增高架 (Autodesk Fusion 360 design; units mm, degrees)
part number: 2026-05-03-09-00-51-112
Autodesk Fusion 360 part; units mm, degrees
(part 1 of 4)
sketch "草图1" plane through (0, 0, 0) normal (0, 0, 1) x (1, 0, 0)
  line L0 (62.5, -90) -> (62.5, 85) construction
  line L1 (57.5, 90) -> (-57.5, 90) construction
  line L2 (-62.5, 85) -> (-62.5, -90) construction
  line L3 (-62.5, -90) -> (62.5, 90) construction
  line L4 (62.5, -90) -> (-62.5, 90) construction
  arc A0 (-57.5, 90) -> (-62.5, 85) centre (-57.5, 85) ccw construction
  arc A1 (62.5, 85) -> (57.5, 90) centre (57.5, 85) ccw construction
  line L5 (64, -90) -> (64, 85)
  arc A2 (64, 85) -> (57.5, 91.5) centre (57.5, 85) ccw
  line L6 (57.5, 91.5) -> (-57.5, 91.5)
  arc A3 (-57.5, 91.5) -> (-64, 85) centre (-57.5, 85) ccw
  line L7 (-64, 85) -> (-64, -90)
  line L8 (61, -90) -> (61, 85)
  arc A4 (61, 85) -> (57.5, 88.5) centre (57.5, 85) ccw
  line L9 (57.5, 88.5) -> (-57.5, 88.5)
  arc A5 (-57.5, 88.5) -> (-61, 85) centre (-57.5, 85) ccw
  line L10 (-61, 85) -> (-61, -90)
  line L11 (-64, -90) -> (-61, -90)
  line L12 (61, -90) -> (64, -90)
  line L13 (60.2436, 25.7321) -> (68.9038, 20.7321)
  dimension "d1" = 125
  dimension "d3" = 180
  dimension "d4" = 5
  dimension "d5" = 5
  dimension "d6" = 1.5
  dimension "d7" = -1.5
  constraint parallel L0 L2
  constraint coincident L3 origin
  constraint coincident L4 origin
  constraint horizontal L1
  constraint vertical L2
  constraint coincident L4.end L1
  constraint coincident L4.end L2
  constraint tangent L1 A0
  constraint tangent L2 A0
  constraint coincident L3.end L1
  constraint coincident L3.end L0
  constraint tangent L1 A1
  constraint tangent L0 A1
  constraint perpendicular L10 L11
  constraint perpendicular L5 L12
  measures "d1" distance of L0 L2
  measures "d3" distance of L2.end L4.end
  measures "d4" radius of A0
  measures "d5" radius of A1
extrude "拉伸1" add sketch "草图1" along normal blind 250
sketch "草图4" plane through (0, 91.5, 0) normal (0, 1, 0) x (-1, 0, 0)
  line L0 (-57.5, 0) -> (57.5, 0)
  line L1 (57.5, 0) -> (57.5, 250)
  line L2 (57.5, 250) -> (-57.5, 250)
  line L3 (-57.5, 250) -> (-57.5, 0)
  line L4 (48.5, 14) -> (44.1699, 11.5)
  line L5 (44.1699, 11.5) -> (44.1699, 6.5)
  line L6 (44.1699, 6.5) -> (48.5, 4)
  line L7 (48.5, 4) -> (52.8301, 6.5)
  line L8 (52.8301, 6.5) -> (52.8301, 11.5)
  line L9 (52.8301, 11.5) -> (48.5, 14)
  line L10 (37.8397, 14) -> (33.5096, 11.5)
  line L11 (33.5096, 11.5) -> (33.5096, 6.5)
  line L12 (33.5096, 6.5) -> (37.8397, 4)
  line L13 (37.8397, 4) -> (42.1699, 6.5)
  line L14 (42.1699, 6.5) -> (42.1699, 11.5)
  line L15 (42.1699, 11.5) -> (37.8397, 14)
  line L16 (27.1795, 14) -> (22.8494, 11.5)
  line L17 (22.8494, 11.5) -> (22.8494, 6.5)
  line L18 (22.8494, 6.5) -> (27.1795, 4)
  line L19 (27.1795, 4) -> (31.5096, 6.5)
  line L20 (31.5096, 6.5) -> (31.5096, 11.5)
  line L21 (31.5096, 11.5) -> (27.1795, 14)
  line L22 (16.5192, 14) -> (12.1891, 11.5)
  line L23 (12.1891, 11.5) -> (12.1891, 6.5)
  line L24 (12.1891, 6.5) -> (16.5192, 4)
  line L25 (16.5192, 4) -> (20.8494, 6.5)
  line L26 (20.8494, 6.5) -> (20.8494, 11.5)
  line L27 (20.8494, 11.5) -> (16.5192, 14)
  line L28 (5.859, 14) -> (1.5289, 11.5)
  line L29 (1.5289, 11.5) -> (1.5289, 6.5)
  line L30 (1.5289, 6.5) -> (5.859, 4)
  line L31 (5.859, 4) -> (10.1891, 6.5)
  line L32 (10.1891, 6.5) -> (10.1891, 11.5)
  line L33 (10.1891, 11.5) -> (5.859, 14)
  line L34 (-4.8013, 14) -> (-9.1314, 11.5)
  line L35 (-9.1314, 11.5) -> (-9.1314, 6.5)
  line L36 (-9.1314, 6.5) -> (-4.8013, 4)
  line L37 (-4.8013, 4) -> (-0.4711, 6.5)
  line L38 (-0.4711, 6.5) -> (-0.4711, 11.5)
  line L39 (-0.4711, 11.5) -> (-4.8013, 14)
  line L40 (-15.4615, 14) -> (-19.7917, 11.5)
  line L41 (-19.7917, 11.5) -> (-19.7917, 6.5)
  line L42 (-19.7917, 6.5) -> (-15.4615, 4)
  line L43 (-15.4615, 4) -> (-11.1314, 6.5)
  line L44 (-11.1314, 6.5) -> (-11.1314, 11.5)
  line L45 (-11.1314, 11.5) -> (-15.4615, 14)
  line L46 (-26.1218, 14) -> (-30.4519, 11.5)
  line L47 (-30.4519, 11.5) -> (-30.4519, 6.5)
  line L48 (-30.4519, 6.5) -> (-26.1218, 4)
  line L49 (-26.1218, 4) -> (-21.7917, 6.5)
  line L50 (-21.7917, 6.5) -> (-21.7917, 11.5)
  line L51 (-21.7917, 11.5) -> (-26.1218, 14)
  line L52 (-36.782, 14) -> (-41.1122, 11.5)
  line L53 (-41.1122, 11.5) -> (-41.1122, 6.5)
  line L54 (-41.1122, 6.5) -> (-36.782, 4)
  line L55 (-36.782, 4) -> (-32.4519, 6.5)
  line L56 (-32.4519, 6.5) -> (-32.4519, 11.5)
  line L57 (-32.4519, 11.5) -> (-36.782, 14)
  line L58 (-47.4423, 14) -> (-51.7724, 11.5)
  line L59 (-51.7724, 11.5) -> (-51.7724, 6.5)
  line L60 (-51.7724, 6.5) -> (-47.4423, 4)
  line L61 (-47.4423, 4) -> (-43.1122, 6.5)
  line L62 (-43.1122, 6.5) -> (-43.1122, 11.5)
  line L63 (-43.1122, 11.5) -> (-47.4423, 14)
  line L64 (43.1699, 23.2321) -> (38.8397, 20.7321)
  line L65 (38.8397, 20.7321) -> (38.8397, 15.7321)
  line L66 (38.8397, 15.7321) -> (43.1699, 13.2321)
  line L67 (43.1699, 13.2321) -> (47.5, 15.7321)
  line L68 (47.5, 15.7321) -> (47.5, 20.7321)
  line L69 (47.5, 20.7321) -> (43.1699, 23.2321)
  line L70 (32.5096, 23.2321) -> (28.1795, 20.7321)
  line L71 (28.1795, 20.7321) -> (28.1795, 15.7321)
  line L72 (28.1795, 15.7321) -> (32.5096, 13.2321)
  line L73 (32.5096, 13.2321) -> (36.8397, 15.7321)
  line L74 (36.8397, 15.7321) -> (36.8397, 20.7321)
  line L75 (36.8397, 20.7321) -> (32.5096, 23.2321)
  line L76 (21.8494, 23.2321) -> (17.5192, 20.7321)
  line L77 (17.5192, 20.7321) -> (17.5192, 15.7321)
  line L78 (17.5192, 15.7321) -> (21.8494, 13.2321)
  line L79 (21.8494, 13.2321) -> (26.1795, 15.7321)
  line L80 (26.1795, 15.7321) -> (26.1795, 20.7321)
  line L81 (26.1795, 20.7321) -> (21.8494, 23.2321)
  line L82 (11.1891, 23.2321) -> (6.859, 20.7321)
  line L83 (6.859, 20.7321) -> (6.859, 15.7321)
  line L84 (6.859, 15.7321) -> (11.1891, 13.2321)
  line L85 (11.1891, 13.2321) -> (15.5192, 15.7321)
  line L86 (15.5192, 15.7321) -> (15.5192, 20.7321)
  line L87 (15.5192, 20.7321) -> (11.1891, 23.2321)
  line L88 (0.5289, 23.2321) -> (-3.8013, 20.7321)
  line L89 (-3.8013, 20.7321) -> (-3.8013, 15.7321)
  line L90 (-3.8013, 15.7321) -> (0.5289, 13.2321)
  line L91 (0.5289, 13.2321) -> (4.859, 15.7321)
  line L92 (4.859, 15.7321) -> (4.859, 20.7321)
  line L93 (4.859, 20.7321) -> (0.5289, 23.2321)
  line L94 (-10.1314, 23.2321) -> (-14.4615, 20.7321)
  line L95 (-14.4615, 20.7321) -> (-14.4615, 15.7321)
  line L96 (-14.4615, 15.7321) -> (-10.1314, 13.2321)
  line L97 (-10.1314, 13.2321) -> (-5.8013, 15.7321)
  line L98 (-5.8013, 15.7321) -> (-5.8013, 20.7321)
  line L99 (-5.8013, 20.7321) -> (-10.1314, 23.2321)
  line L100 (-20.7917, 23.2321) -> (-25.1218, 20.7321)
  line L101 (-25.1218, 20.7321) -> (-25.1218, 15.7321)
  line L102 (-25.1218, 15.7321) -> (-20.7917, 13.2321)
  line L103 (-20.7917, 13.2321) -> (-16.4615, 15.7321)
  line L104 (-16.4615, 15.7321) -> (-16.4615, 20.7321)
  line L105 (-16.4615, 20.7321) -> (-20.7917, 23.2321)
  line L106 (-31.4519, 23.2321) -> (-35.782, 20.7321)
  line L107 (-35.782, 20.7321) -> (-35.782, 15.7321)
  line L108 (-35.782, 15.7321) -> (-31.4519, 13.2321)
  line L109 (-31.4519, 13.2321) -> (-27.1218, 15.7321)
  line L110 (-27.1218, 15.7321) -> (-27.1218, 20.7321)
  line L111 (-27.1218, 20.7321) -> (-31.4519, 23.2321)
  line L112 (-42.1122, 23.2321) -> (-46.4423, 20.7321)
  line L113 (-46.4423, 20.7321) -> (-46.4423, 15.7321)
  line L114 (-46.4423, 15.7321) -> (-42.1122, 13.2321)
  line L115 (-42.1122, 13.2321) -> (-37.782, 15.7321)
  line L116 (-37.782, 15.7321) -> (-37.782, 20.7321)
  line L117 (-37.782, 20.7321) -> (-42.1122, 23.2321)
  line L118 (48.5, 32.4641) -> (44.1699, 29.9641)
  line L119 (44.1699, 29.9641) -> (44.1699, 24.9641)
  line L120 (44.1699, 24.9641) -> (48.5, 22.4641)
  line L121 (48.5, 22.4641) -> (52.8301, 24.9641)
  line L122 (52.8301, 24.9641) -> (52.8301, 29.9641)
  line L123 (52.8301, 29.9641) -> (48.5, 32.4641)
  line L124 (37.8397, 32.4641) -> (33.5096, 29.9641)
  line L125 (33.5096, 29.9641) -> (33.5096, 24.9641)
  line L126 (33.5096, 24.9641) -> (37.8397, 22.4641)
  line L127 (37.8397, 22.4641) -> (42.1699, 24.9641)
  line L128 (42.1699, 24.9641) -> (42.1699, 29.9641)
  line L129 (42.1699, 29.9641) -> (37.8397, 32.4641)
  line L130 (27.1795, 32.4641) -> (22.8494, 29.9641)
  line L131 (22.8494, 29.9641) -> (22.8494, 24.9641)
  line L132 (22.8494, 24.9641) -> (27.1795, 22.4641)
  line L133 (27.1795, 22.4641) -> (31.5096, 24.9641)
  line L134 (31.5096, 24.9641) -> (31.5096, 29.9641)
  line L135 (31.5096, 29.9641) -> (27.1795, 32.4641)
  line L136 (16.5192, 32.4641) -> (12.1891, 29.9641)
  line L137 (12.1891, 29.9641) -> (12.1891, 24.9641)
  line L138 (12.1891, 24.9641) -> (16.5192, 22.4641)
  line L139 (16.5192, 22.4641) -> (20.8494, 24.9641)
  line L140 (20.8494, 24.9641) -> (20.8494, 29.9641)
  line L141 (20.8494, 29.9641) -> (16.5192, 32.4641)
  line L142 (5.859, 32.4641) -> (1.5289, 29.9641)
  line L143 (1.5289, 29.9641) -> (1.5289, 24.9641)
  line L144 (1.5289, 24.9641) -> (5.859, 22.4641)
  line L145 (5.859, 22.4641) -> (10.1891, 24.9641)
  line L146 (10.1891, 24.9641) -> (10.1891, 29.9641)
  line L147 (10.1891, 29.9641) -> (5.859, 32.4641)
  line L148 (-4.8013, 32.4641) -> (-9.1314, 29.9641)
  line L149 (-9.1314, 29.9641) -> (-9.1314, 24.9641)
  line L150 (-9.1314, 24.9641) -> (-4.8013, 22.4641)
  line L151 (-4.8013, 22.4641) -> (-0.4711, 24.9641)
  line L152 (-0.4711, 24.9641) -> (-0.4711, 29.9641)
  line L153 (-0.4711, 29.9641) -> (-4.8013, 32.4641)
  line L154 (-15.4615, 32.4641) -> (-19.7917, 29.9641)
  line L155 (-19.7917, 29.9641) -> (-19.7917, 24.9641)
  line L156 (-19.7917, 24.9641) -> (-15.4615, 22.4641)
  line L157 (-15.4615, 22.4641) -> (-11.1314, 24.9641)
  line L158 (-11.1314, 24.9641) -> (-11.1314, 29.9641)
  line L159 (-11.1314, 29.9641) -> (-15.4615, 32.4641)
  line L160 (-26.1218, 32.4641) -> (-30.4519, 29.9641)
  line L161 (-30.4519, 29.9641) -> (-30.4519, 24.9641)
  line L162 (-30.4519, 24.9641) -> (-26.1218, 22.4641)
  line L163 (-26.1218, 22.4641) -> (-21.7917, 24.9641)
  line L164 (-21.7917, 24.9641) -> (-21.7917, 29.9641)
  line L165 (-21.7917, 29.9641) -> (-26.1218, 32.4641)
  line L166 (-36.782, 32.4641) -> (-41.1122, 29.9641)
  line L167 (-41.1122, 29.9641) -> (-41.1122, 24.9641)
  line L168 (-41.1122, 24.9641) -> (-36.782, 22.4641)
  line L169 (-36.782, 22.4641) -> (-32.4519, 24.9641)
  line L170 (-32.4519, 24.9641) -> (-32.4519, 29.9641)
  line L171 (-32.4519, 29.9641) -> (-36.782, 32.4641)
  line L172 (-47.4423, 32.4641) -> (-51.7724, 29.9641)
  line L173 (-51.7724, 29.9641) -> (-51.7724, 24.9641)
  line L174 (-51.7724, 24.9641) -> (-47.4423, 22.4641)
  line L175 (-47.4423, 22.4641) -> (-43.1122, 24.9641)
  line L176 (-43.1122, 24.9641) -> (-43.1122, 29.9641)
  line L177 (-43.1122, 29.9641) -> (-47.4423, 32.4641)
  line L178 (43.1699, 41.6962) -> (38.8397, 39.1962)
  line L179 (38.8397, 39.1962) -> (38.8397, 34.1962)
  line L180 (38.8397, 34.1962) -> (43.1699, 31.6962)
  line L181 (43.1699, 31.6962) -> (47.5, 34.1962)
  line L182 (47.5, 34.1962) -> (47.5, 39.1962)
  line L183 (47.5, 39.1962) -> (43.1699, 41.6962)
  line L184 (32.5096, 41.6962) -> (28.1795, 39.1962)
  line L185 (28.1795, 39.1962) -> (28.1795, 34.1962)
  line L186 (28.1795, 34.1962) -> (32.5096, 31.6962)
  line L187 (32.5096, 31.6962) -> (36.8397, 34.1962)
  line L188 (36.8397, 34.1962) -> (36.8397, 39.1962)
  line L189 (36.8397, 39.1962) -> (32.5096, 41.6962)
  line L190 (21.8494, 41.6962) -> (17.5192, 39.1962)
  line L191 (17.5192, 39.1962) -> (17.5192, 34.1962)
  line L192 (17.5192, 34.1962) -> (21.8494, 31.6962)
  line L193 (21.8494, 31.6962) -> (26.1795, 34.1962)
  line L194 (26.1795, 34.1962) -> (26.1795, 39.1962)
  line L195 (26.1795, 39.1962) -> (21.8494, 41.6962)
  line L196 (11.1891, 41.6962) -> (6.859, 39.1962)
  line L197 (6.859, 39.1962) -> (6.859, 34.1962)
  line L198 (6.859, 34.1962) -> (11.1891, 31.6962)
  line L199 (11.1891, 31.6962) -> (15.5192, 34.1962)
  line L200 (15.5192, 34.1962) -> (15.5192, 39.1962)
  line L201 (15.5192, 39.1962) -> (11.1891, 41.6962)
  line L202 (0.5289, 41.6962) -> (-3.8013, 39.1962)
  line L203 (-3.8013, 39.1962) -> (-3.8013, 34.1962)
  line L204 (-3.8013, 34.1962) -> (0.5289, 31.6962)
  line L205 (0.5289, 31.6962) -> (4.859, 34.1962)
  line L206 (4.859, 34.1962) -> (4.859, 39.1962)
  line L207 (4.859, 39.1962) -> (0.5289, 41.6962)
  line L208 (-10.1314, 41.6962) -> (-14.4615, 39.1962)
  line L209 (-14.4615, 39.1962) -> (-14.4615, 34.1962)
  line L210 (-14.4615, 34.1962) -> (-10.1314, 31.6962)
  line L211 (-10.1314, 31.6962) -> (-5.8013, 34.1962)
  line L212 (-5.8013, 34.1962) -> (-5.8013, 39.1962)
  line L213 (-5.8013, 39.1962) -> (-10.1314, 41.6962)
  line L214 (-20.7917, 41.6962) -> (-25.1218, 39.1962)
  line L215 (-25.1218, 39.1962) -> (-25.1218, 34.1962)
  line L216 (-25.1218, 34.1962) -> (-20.7917, 31.6962)
  line L217 (-20.7917, 31.6962) -> (-16.4615, 34.1962)
  line L218 (-16.4615, 34.1962) -> (-16.4615, 39.1962)
  line L219 (-16.4615, 39.1962) -> (-20.7917, 41.6962)
  line L220 (-31.4519, 41.6962) -> (-35.782, 39.1962)
  line L221 (-35.782, 39.1962) -> (-35.782, 34.1962)
  line L222 (-35.782, 34.1962) -> (-31.4519, 31.6962)
  line L223 (-31.4519, 31.6962) -> (-27.1218, 34.1962)
  line L224 (-27.1218, 34.1962) -> (-27.1218, 39.1962)
  line L225 (-27.1218, 39.1962) -> (-31.4519, 41.6962)
  line L226 (-42.1122, 41.6962) -> (-46.4423, 39.1962)
  line L227 (-46.4423, 39.1962) -> (-46.4423, 34.1962)
  line L228 (-46.4423, 34.1962) -> (-42.1122, 31.6962)
  line L229 (-42.1122, 31.6962) -> (-37.782, 34.1962)
  line L230 (-37.782, 34.1962) -> (-37.782, 39.1962)
  line L231 (-37.782, 39.1962) -> (-42.1122, 41.6962)
  line L232 (48.5, 50.9282) -> (44.1699, 48.4282)
  line L233 (44.1699, 48.4282) -> (44.1699, 43.4282)
  line L234 (44.1699, 43.4282) -> (48.5, 40.9282)
  line L235 (48.5, 40.9282) -> (52.8301, 43.4282)
  line L236 (52.8301, 43.4282) -> (52.8301, 48.4282)
  line L237 (52.8301, 48.4282) -> (48.5, 50.9282)
  line L238 (37.8397, 50.9282) -> (33.5096, 48.4282)
  line L239 (33.5096, 48.4282) -> (33.5096, 43.4282)
  line L240 (33.5096, 43.4282) -> (37.8397, 40.9282)
  line L241 (37.8397, 40.9282) -> (42.1699, 43.4282)
  line L242 (42.1699, 43.4282) -> (42.1699, 48.4282)
  line L243 (42.1699, 48.4282) -> (37.8397, 50.9282)
  line L244 (27.1795, 50.9282) -> (22.8494, 48.4282)
  line L245 (22.8494, 48.4282) -> (22.8494, 43.4282)
  line L246 (22.8494, 43.4282) -> (27.1795, 40.9282)
  line L247 (27.1795, 40.9282) -> (31.5096, 43.4282)
  line L248 (31.5096, 43.4282) -> (31.5096, 48.4282)
  line L249 (31.5096, 48.4282) -> (27.1795, 50.9282)
  line L250 (16.5192, 50.9282) -> (12.1891, 48.4282)
  line L251 (12.1891, 48.4282) -> (12.1891, 43.4282)
  line L252 (12.1891, 43.4282) -> (16.5192, 40.9282)
  line L253 (16.5192, 40.9282) -> (20.8494, 43.4282)
  line L254 (20.8494, 43.4282) -> (20.8494, 48.4282)
  line L255 (20.8494, 48.4282) -> (16.5192, 50.9282)
  line L256 (5.859, 50.9282) -> (1.5289, 48.4282)
  line L257 (1.5289, 48.4282) -> (1.5289, 43.4282)
  line L258 (1.5289, 43.4282) -> (5.859, 40.9282)
  line L259 (5.859, 40.9282) -> (10.1891, 43.4282)
  line L260 (10.1891, 43.4282) -> (10.1891, 48.4282)
  line L261 (10.1891, 48.4282) -> (5.859, 50.9282)
  line L262 (-4.8013, 50.9282) -> (-9.1314, 48.4282)
  line L263 (-9.1314, 48.4282) -> (-9.1314, 43.4282)
  line L264 (-9.1314, 43.4282) -> (-4.8013, 40.9282)
  line L265 (-4.8013, 40.9282) -> (-0.4711, 43.4282)
  line L266 (-0.4711, 43.4282) -> (-0.4711, 48.4282)
  line L267 (-0.4711, 48.4282) -> (-4.8013, 50.9282)
  line L268 (-15.4615, 50.9282) -> (-19.7917, 48.4282)
  line L269 (-19.7917, 48.4282) -> (-19.7917, 43.4282)
  line L270 (-19.7917, 43.4282) -> (-15.4615, 40.9282)
  line L271 (-15.4615, 40.9282) -> (-11.1314, 43.4282)
  line L272 (-11.1314, 43.4282) -> (-11.1314, 48.4282)
  line L273 (-11.1314, 48.4282) -> (-15.4615, 50.9282)
  line L274 (-26.1218, 50.9282) -> (-30.4519, 48.4282)
  line L275 (-30.4519, 48.4282) -> (-30.4519, 43.4282)
  line L276 (-30.4519, 43.4282) -> (-26.1218, 40.9282)
  line L277 (-26.1218, 40.9282) -> (-21.7917, 43.4282)
  line L278 (-21.7917, 43.4282) -> (-21.7917, 48.4282)
  line L279 (-21.7917, 48.4282) -> (-26.1218, 50.9282)
  line L280 (-36.782, 50.9282) -> (-41.1122, 48.4282)
  line L281 (-41.1122, 48.4282) -> (-41.1122, 43.4282)
  line L282 (-41.1122, 43.4282) -> (-36.782, 40.9282)
  line L283 (-36.782, 40.9282) -> (-32.4519, 43.4282)
  line L284 (-32.4519, 43.4282) -> (-32.4519, 48.4282)
  line L285 (-32.4519, 48.4282) -> (-36.782, 50.9282)
  line L286 (-47.4423, 50.9282) -> (-51.7724, 48.4282)
  line L287 (-51.7724, 48.4282) -> (-51.7724, 43.4282)
  line L288 (-51.7724, 43.4282) -> (-47.4423, 40.9282)
  line L289 (-47.4423, 40.9282) -> (-43.1122, 43.4282)
  line L290 (-43.1122, 43.4282) -> (-43.1122, 48.4282)
  line L291 (-43.1122, 48.4282) -> (-47.4423, 50.9282)
  line L292 (43.1699, 60.1603) -> (38.8397, 57.6603)
  line L293 (38.8397, 57.6603) -> (38.8397, 52.6603)
  line L294 (38.8397, 52.6603) -> (43.1699, 50.1603)
  line L295 (43.1699, 50.1603) -> (47.5, 52.6603)
  line L296 (47.5, 52.6603) -> (47.5, 57.6603)
  line L297 (47.5, 57.6603) -> (43.1699, 60.1603)
  line L298 (32.5096, 60.1603) -> (28.1795, 57.6603)
  line L299 (28.1795, 57.6603) -> (28.1795, 52.6603)
  line L300 (28.1795, 52.6603) -> (32.5096, 50.1603)
  line L301 (32.5096, 50.1603) -> (36.8397, 52.6603)
  line L302 (36.8397, 52.6603) -> (36.8397, 57.6603)
  line L303 (36.8397, 57.6603) -> (32.5096, 60.1603)
  line L304 (21.8494, 60.1603) -> (17.5192, 57.6603)
  line L305 (17.5192, 57.6603) -> (17.5192, 52.6603)
  line L306 (17.5192, 52.6603) -> (21.8494, 50.1603)
  line L307 (21.8494, 50.1603) -> (26.1795, 52.6603)
  line L308 (26.1795, 52.6603) -> (26.1795, 57.6603)
  line L309 (26.1795, 57.6603) -> (21.8494, 60.1603)
  line L310 (11.1891, 60.1603) -> (6.859, 57.6603)
  line L311 (6.859, 57.6603) -> (6.859, 52.6603)
  line L312 (6.859, 52.6603) -> (11.1891, 50.1603)
  line L313 (11.1891, 50.1603) -> (15.5192, 52.6603)
  line L314 (15.5192, 52.6603) -> (15.5192, 57.6603)
  line L315 (15.5192, 57.6603) -> (11.1891, 60.1603)
  line L316 (0.5289, 60.1603) -> (-3.8013, 57.6603)
  line L317 (-3.8013, 57.6603) -> (-3.8013, 52.6603)
  line L318 (-3.8013, 52.6603) -> (0.5289, 50.1603)
  line L319 (0.5289, 50.1603) -> (4.859, 52.6603)
  line L320 (4.859, 52.6603) -> (4.859, 57.6603)
  line L321 (4.859, 57.6603) -> (0.5289, 60.1603)
  line L322 (-10.1314, 60.1603) -> (-14.4615, 57.6603)
  line L323 (-14.4615, 57.6603) -> (-14.4615, 52.6603)
  line L324 (-14.4615, 52.6603) -> (-10.1314, 50.1603)
  line L325 (-10.1314, 50.1603) -> (-5.8013, 52.6603)
  line L326 (-5.8013, 52.6603) -> (-5.8013, 57.6603)
  line L327 (-5.8013, 57.6603) -> (-10.1314, 60.1603)
  line L328 (-20.7917, 60.1603) -> (-25.1218, 57.6603)
  line L329 (-25.1218, 57.6603) -> (-25.1218, 52.6603)
  line L330 (-25.1218, 52.6603) -> (-20.7917, 50.1603)
  line L331 (-20.7917, 50.1603) -> (-16.4615, 52.6603)
  line L332 (-16.4615, 52.6603) -> (-16.4615, 57.6603)
  line L333 (-16.4615, 57.6603) -> (-20.7917, 60.1603)
  line L334 (-31.4519, 60.1603) -> (-35.782, 57.6603)
  line L335 (-35.782, 57.6603) -> (-35.782, 52.6603)
  line L336 (-35.782, 52.6603) -> (-31.4519, 50.1603)
  line L337 (-31.4519, 50.1603) -> (-27.1218, 52.6603)
  line L338 (-27.1218, 52.6603) -> (-27.1218, 57.6603)
  line L339 (-27.1218, 57.6603) -> (-31.4519, 60.1603)
  line L340 (-42.1122, 60.1603) -> (-46.4423, 57.6603)
  line L341 (-46.4423, 57.6603) -> (-46.4423, 52.6603)
  line L342 (-46.4423, 52.6603) -> (-42.1122, 50.1603)
  line L343 (-42.1122, 50.1603) -> (-37.782, 52.6603)
  line L344 (-37.782, 52.6603) -> (-37.782, 57.6603)
  line L345 (-37.782, 57.6603) -> (-42.1122, 60.1603)
  line L346 (48.5, 69.3923) -> (44.1699, 66.8923)
  line L347 (44.1699, 66.8923) -> (44.1699, 61.8923)
  line L348 (44.1699, 61.8923) -> (48.5, 59.3923)
  line L349 (48.5, 59.3923) -> (52.8301, 61.8923)
  line L350 (52.8301, 61.8923) -> (52.8301, 66.8923)
  line L351 (52.8301, 66.8923) -> (48.5, 69.3923)
  line L352 (37.8397, 69.3923) -> (33.5096, 66.8923)
  line L353 (33.5096, 66.8923) -> (33.5096, 61.8923)
  line L354 (33.5096, 61.8923) -> (37.8397, 59.3923)
  line L355 (37.8397, 59.3923) -> (42.1699, 61.8923)
  line L356 (42.1699, 61.8923) -> (42.1699, 66.8923)
  line L357 (42.1699, 66.8923) -> (37.8397, 69.3923)
  line L358 (27.1795, 69.3923) -> (22.8494, 66.8923)
  line L359 (22.8494, 66.8923) -> (22.8494, 61.8923)
  line L360 (22.8494, 61.8923) -> (27.1795, 59.3923)
  line L361 (27.1795, 59.3923) -> (31.5096, 61.8923)
  line L362 (31.5096, 61.8923) -> (31.5096, 66.8923)
  line L363 (31.5096, 66.8923) -> (27.1795, 69.3923)
  line L364 (16.5192, 69.3923) -> (12.1891, 66.8923)
  line L365 (12.1891, 66.8923) -> (12.1891, 61.8923)
  line L366 (12.1891, 61.8923) -> (16.5192, 59.3923)
  line L367 (16.5192, 59.3923) -> (20.8494, 61.8923)
  line L368 (20.8494, 61.8923) -> (20.8494, 66.8923)
  line L369 (20.8494, 66.8923) -> (16.5192, 69.3923)
  line L370 (5.859, 69.3923) -> (1.5289, 66.8923)
  line L371 (1.5289, 66.8923) -> (1.5289, 61.8923)
  line L372 (1.5289, 61.8923) -> (5.859, 59.3923)
  line L373 (5.859, 59.3923) -> (10.1891, 61.8923)
  line L374 (10.1891, 61.8923) -> (10.1891, 66.8923)
  line L375 (10.1891, 66.8923) -> (5.859, 69.3923)
  line L376 (-4.8013, 69.3923) -> (-9.1314, 66.8923)
  line L377 (-9.1314, 66.8923) -> (-9.1314, 61.8923)
  line L378 (-9.1314, 61.8923) -> (-4.8013, 59.3923)
  line L379 (-4.8013, 59.3923) -> (-0.4711, 61.8923)
  line L380 (-0.4711, 61.8923) -> (-0.4711, 66.8923)
  line L381 (-0.4711, 66.8923) -> (-4.8013, 69.3923)
  line L382 (-15.4615, 69.3923) -> (-19.7917, 66.8923)
  line L383 (-19.7917, 66.8923) -> (-19.7917, 61.8923)
  line L384 (-19.7917, 61.8923) -> (-15.4615, 59.3923)
  line L385 (-15.4615, 59.3923) -> (-11.1314, 61.8923)
  line L386 (-11.1314, 61.8923) -> (-11.1314, 66.8923)
  line L387 (-11.1314, 66.8923) -> (-15.4615, 69.3923)
  line L388 (-26.1218, 69.3923) -> (-30.4519, 66.8923)
  line L389 (-30.4519, 66.8923) -> (-30.4519, 61.8923)
  line L390 (-30.4519, 61.8923) -> (-26.1218, 59.3923)
  line L391 (-26.1218, 59.3923) -> (-21.7917, 61.8923)
  line L392 (-21.7917, 61.8923) -> (-21.7917, 66.8923)
  line L393 (-21.7917, 66.8923) -> (-26.1218, 69.3923)
  line L394 (-36.782, 69.3923) -> (-41.1122, 66.8923)
  line L395 (-41.1122, 66.8923) -> (-41.1122, 61.8923)
  line L396 (-41.1122, 61.8923) -> (-36.782, 59.3923)
  line L397 (-36.782, 59.3923) -> (-32.4519, 61.8923)
  line L398 (-32.4519, 61.8923) -> (-32.4519, 66.8923)
  line L399 (-32.4519, 66.8923) -> (-36.782, 69.3923)
  line L400 (-47.4423, 69.3923) -> (-51.7724, 66.8923)
  line L401 (-51.7724, 66.8923) -> (-51.7724, 61.8923)
  line L402 (-51.7724, 61.8923) -> (-47.4423, 59.3923)
  line L403 (-47.4423, 59.3923) -> (-43.1122, 61.8923)
  line L404 (-43.1122, 61.8923) -> (-43.1122, 66.8923)
  line L405 (-43.1122, 66.8923) -> (-47.4423, 69.3923)
  line L406 (43.1699, 78.6244) -> (38.8397, 76.1244)
  line L407 (38.8397, 76.1244) -> (38.8397, 71.1244)
  line L408 (38.8397, 71.1244) -> (43.1699, 68.6244)
  line L409 (43.1699, 68.6244) -> (47.5, 71.1244)
  line L410 (47.5, 71.1244) -> (47.5, 76.1244)
  line L411 (47.5, 76.1244) -> (43.1699, 78.6244)
  line L412 (32.5096, 78.6244) -> (28.1795, 76.1244)
  line L413 (28.1795, 76.1244) -> (28.1795, 71.1244)
  line L414 (28.1795, 71.1244) -> (32.5096, 68.6244)
  line L415 (32.5096, 68.6244) -> (36.8397, 71.1244)
  line L416 (36.8397, 71.1244) -> (36.8397, 76.1244)
  line L417 (36.8397, 76.1244) -> (32.5096, 78.6244)
  line L418 (21.8494, 78.6244) -> (17.5192, 76.1244)
  line L419 (17.5192, 76.1244) -> (17.5192, 71.1244)
  line L420 (17.5192, 71.1244) -> (21.8494, 68.6244)
  line L421 (21.8494, 68.6244) -> (26.1795, 71.1244)
  line L422 (26.1795, 71.1244) -> (26.1795, 76.1244)
  line L423 (26.1795, 76.1244) -> (21.8494, 78.6244)
  line L424 (11.1891, 78.6244) -> (6.859, 76.1244)
  line L425 (6.859, 76.1244) -> (6.859, 71.1244)
  line L426 (6.859, 71.1244) -> (11.1891, 68.6244)
  line L427 (11.1891, 68.6244) -> (15.5192, 71.1244)
  line L428 (15.5192, 71.1244) -> (15.5192, 76.1244)
  line L429 (15.5192, 76.1244) -> (11.1891, 78.6244)
  line L430 (0.5289, 78.6244) -> (-3.8013, 76.1244)
  line L431 (-3.8013, 76.1244) -> (-3.8013, 71.1244)
  line L432 (-3.8013, 71.1244) -> (0.5289, 68.6244)
  line L433 (0.5289, 68.6244) -> (4.859, 71.1244)
  line L434 (4.859, 71.1244) -> (4.859, 76.1244)
  line L435 (4.859, 76.1244) -> (0.5289, 78.6244)
  line L436 (-10.1314, 78.6244) -> (-14.4615, 76.1244)
  line L437 (-14.4615, 76.1244) -> (-14.4615, 71.1244)
  line L438 (-14.4615, 71.1244) -> (-10.1314, 68.6244)
  line L439 (-10.1314, 68.6244) -> (-5.8013, 71.1244)
  line L440 (-5.8013, 71.1244) -> (-5.8013, 76.1244)
  line L441 (-5.8013, 76.1244) -> (-10.1314, 78.6244)
  line L442 (-20.7917, 78.6244) -> (-25.1218, 76.1244)
  line L443 (-25.1218, 76.1244) -> (-25.1218, 71.1244)
  line L444 (-25.1218, 71.1244) -> (-20.7917, 68.6244)
  line L445 (-20.7917, 68.6244) -> (-16.4615, 71.1244)
  line L446 (-16.4615, 71.1244) -> (-16.4615, 76.1244)
  line L447 (-16.4615, 76.1244) -> (-20.7917, 78.6244)
  line L448 (-31.4519, 78.6244) -> (-35.782, 76.1244)
  line L449 (-35.782, 76.1244) -> (-35.782, 71.1244)
  line L450 (-35.782, 71.1244) -> (-31.4519, 68.6244)
  line L451 (-31.4519, 68.6244) -> (-27.1218, 71.1244)
  line L452 (-27.1218, 71.1244) -> (-27.1218, 76.1244)
  line L453 (-27.1218, 76.1244) -> (-31.4519, 78.6244)
  line L454 (-42.1122, 78.6244) -> (-46.4423, 76.1244)
  line L455 (-46.4423, 76.1244) -> (-46.4423, 71.1244)
  line L456 (-46.4423, 71.1244) -> (-42.1122, 68.6244)
  line L457 (-42.1122, 68.6244) -> (-37.782, 71.1244)
  line L458 (-37.782, 71.1244) -> (-37.782, 76.1244)
  line L459 (-37.782, 76.1244) -> (-42.1122, 78.6244)
  line L460 (48.5, 87.8564) -> (44.1699, 85.3564)
  line L461 (44.1699, 85.3564) -> (44.1699, 80.3564)
  line L462 (44.1699, 80.3564) -> (48.5, 77.8564)
  line L463 (48.5, 77.8564) -> (52.8301, 80.3564)
  line L464 (52.8301, 80.3564) -> (52.8301, 85.3564)
  line L465 (52.8301, 85.3564) -> (48.5, 87.8564)
  line L466 (37.8397, 87.8564) -> (33.5096, 85.3564)
  line L467 (33.5096, 85.3564) -> (33.5096, 80.3564)
  line L468 (33.5096, 80.3564) -> (37.8397, 77.8564)
  line L469 (37.8397, 77.8564) -> (42.1699, 80.3564)
  line L470 (42.1699, 80.3564) -> (42.1699, 85.3564)
  line L471 (42.1699, 85.3564) -> (37.8397, 87.8564)
  line L472 (27.1795, 87.8564) -> (22.8494, 85.3564)
  line L473 (22.8494, 85.3564) -> (22.8494, 80.3564)
  line L474 (22.8494, 80.3564) -> (27.1795, 77.8564)
  line L475 (27.1795, 77.8564) -> (31.5096, 80.3564)
  line L476 (31.5096, 80.3564) -> (31.5096, 85.3564)
  line L477 (31.5096, 85.3564) -> (27.1795, 87.8564)
  line L478 (16.5192, 87.8564) -> (12.1891, 85.3564)
  line L479 (12.1891, 85.3564) -> (12.1891, 80.3564)
  line L480 (12.1891, 80.3564) -> (16.5192, 77.8564)
  line L481 (16.5192, 77.8564) -> (20.8494, 80.3564)
  line L482 (20.8494, 80.3564) -> (20.8494, 85.3564)
  line L483 (20.8494, 85.3564) -> (16.5192, 87.8564)
  line L484 (5.859, 87.8564) -> (1.5289, 85.3564)
  line L485 (1.5289, 85.3564) -> (1.5289, 80.3564)
  line L486 (1.5289, 80.3564) -> (5.859, 77.8564)
  line L487 (5.859, 77.8564) -> (10.1891, 80.3564)
  line L488 (10.1891, 80.3564) -> (10.1891, 85.3564)
  line L489 (10.1891, 85.3564) -> (5.859, 87.8564)
  line L490 (-4.8013, 87.8564) -> (-9.1314, 85.3564)
  line L491 (-9.1314, 85.3564) -> (-9.1314, 80.3564)
  line L492 (-9.1314, 80.3564) -> (-4.8013, 77.8564)
  line L493 (-4.8013, 77.8564) -> (-0.4711, 80.3564)
  line L494 (-0.4711, 80.3564) -> (-0.4711, 85.3564)
  line L495 (-0.4711, 85.3564) -> (-4.8013, 87.8564)
  line L496 (-15.4615, 87.8564) -> (-19.7917, 85.3564)
  line L497 (-19.7917, 85.3564) -> (-19.7917, 80.3564)
  line L498 (-19.7917, 80.3564) -> (-15.4615, 77.8564)
  line L499 (-15.4615, 77.8564) -> (-11.1314, 80.3564)
  line L500 (-11.1314, 80.3564) -> (-11.1314, 85.3564)
  line L501 (-11.1314, 85.3564) -> (-15.4615, 87.8564)
  line L502 (-26.1218, 87.8564) -> (-30.4519, 85.3564)
  line L503 (-30.4519, 85.3564) -> (-30.4519, 80.3564)
  line L504 (-30.4519, 80.3564) -> (-26.1218, 77.8564)
  line L505 (-26.1218, 77.8564) -> (-21.7917, 80.3564)
  line L506 (-21.7917, 80.3564) -> (-21.7917, 85.3564)
  line L507 (-21.7917, 85.3564) -> (-26.1218, 87.8564)
  line L508 (-36.782, 87.8564) -> (-41.1122, 85.3564)
  line L509 (-41.1122, 85.3564) -> (-41.1122, 80.3564)
  line L510 (-41.1122, 80.3564) -> (-36.782, 77.8564)
  line L511 (-36.782, 77.8564) -> (-32.4519, 80.3564)
  line L512 (-32.4519, 80.3564) -> (-32.4519, 85.3564)
  line L513 (-32.4519, 85.3564) -> (-36.782, 87.8564)
  line L514 (-47.4423, 87.8564) -> (-51.7724, 85.3564)
  line L515 (-51.7724, 85.3564) -> (-51.7724, 80.3564)
  line L516 (-51.7724, 80.3564) -> (-47.4423, 77.8564)
  line L517 (-47.4423, 77.8564) -> (-43.1122, 80.3564)
  line L518 (-43.1122, 80.3564) -> (-43.1122, 85.3564)
  line L519 (-43.1122, 85.3564) -> (-47.4423, 87.8564)
  line L520 (43.1699, 97.0885) -> (38.8397, 94.5885)
  line L521 (38.8397, 94.5885) -> (38.8397, 89.5885)
  line L522 (38.8397, 89.5885) -> (43.1699, 87.0885)
  line L523 (43.1699, 87.0885) -> (47.5, 89.5885)
  line L524 (47.5, 89.5885) -> (47.5, 94.5885)
  line L525 (47.5, 94.5885) -> (43.1699, 97.0885)
  line L526 (32.5096, 97.0885) -> (28.1795, 94.5885)
  line L527 (28.1795, 94.5885) -> (28.1795, 89.5885)
  line L528 (28.1795, 89.5885) -> (32.5096, 87.0885)
  line L529 (32.5096, 87.0885) -> (36.8397, 89.5885)
  line L530 (36.8397, 89.5885) -> (36.8397, 94.5885)
  line L531 (36.8397, 94.5885) -> (32.5096, 97.0885)
  line L532 (21.8494, 97.0885) -> (17.5192, 94.5885)
  line L533 (17.5192, 94.5885) -> (17.5192, 89.5885)
  line L534 (17.5192, 89.5885) -> (21.8494, 87.0885)
  line L535 (21.8494, 87.0885) -> (26.1795, 89.5885)
  line L536 (26.1795, 89.5885) -> (26.1795, 94.5885)
  line L537 (26.1795, 94.5885) -> (21.8494, 97.0885)
  line L538 (11.1891, 97.0885) -> (6.859, 94.5885)
  line L539 (6.859, 94.5885) -> (6.859, 89.5885)
  line L540 (6.859, 89.5885) -> (11.1891, 87.0885)
  line L541 (11.1891, 87.0885) -> (15.5192, 89.5885)
  line L542 (15.5192, 89.5885) -> (15.5192, 94.5885)
  line L543 (15.5192, 94.5885) -> (11.1891, 97.0885)
  line L544 (0.5289, 97.0885) -> (-3.8013, 94.5885)
  line L545 (-3.8013, 94.5885) -> (-3.8013, 89.5885)
  line L546 (-3.8013, 89.5885) -> (0.5289, 87.0885)
  line L547 (0.5289, 87.0885) -> (4.859, 89.5885)
  line L548 (4.859, 89.5885) -> (4.859, 94.5885)
  line L549 (4.859, 94.5885) -> (0.5289, 97.0885)
  line L550 (-10.1314, 97.0885) -> (-14.4615, 94.5885)
  line L551 (-14.4615, 94.5885) -> (-14.4615, 89.5885)
  line L552 (-14.4615, 89.5885) -> (-10.1314, 87.0885)
  line L553 (-10.1314, 87.0885) -> (-5.8013, 89.5885)
  line L554 (-5.8013, 89.5885) -> (-5.8013, 94.5885)
  line L555 (-5.8013, 94.5885) -> (-10.1314, 97.0885)
  line L556 (-20.7917, 97.0885) -> (-25.1218, 94.5885)
  line L557 (-25.1218, 94.5885) -> (-25.1218, 89.5885)
  line L558 (-25.1218, 89.5885) -> (-20.7917, 87.0885)
  line L559 (-20.7917, 87.0885) -> (-16.4615, 89.5885)
  line L560 (-16.4615, 89.5885) -> (-16.4615, 94.5885)
  line L561 (-16.4615, 94.5885) -> (-20.7917, 97.0885)
  line L562 (-31.4519, 97.0885) -> (-35.782, 94.5885)
  line L563 (-35.782, 94.5885) -> (-35.782, 89.5885)
  line L564 (-35.782, 89.5885) -> (-31.4519, 87.0885)
  line L565 (-31.4519, 87.0885) -> (-27.1218, 89.5885)
  line L566 (-27.1218, 89.5885) -> (-27.1218, 94.5885)
  line L567 (-27.1218, 94.5885) -> (-31.4519, 97.0885)
  line L568 (-42.1122, 97.0885) -> (-46.4423, 94.5885)
  line L569 (-46.4423, 94.5885) -> (-46.4423, 89.5885)
  line L570 (-46.4423, 89.5885) -> (-42.1122, 87.0885)
  line L571 (-42.1122, 87.0885) -> (-37.782, 89.5885)
  line L572 (-37.782, 89.5885) -> (-37.782, 94.5885)
  line L573 (-37.782, 94.5885) -> (-42.1122, 97.0885)
  line L574 (48.5, 106.3205) -> (44.1699, 103.8205)
  line L575 (44.1699, 103.8205) -> (44.1699, 98.8205)
  line L576 (44.1699, 98.8205) -> (48.5, 96.3205)
  line L577 (48.5, 96.3205) -> (52.8301, 98.8205)
  line L578 (52.8301, 98.8205) -> (52.8301, 103.8205)
  line L579 (52.8301, 103.8205) -> (48.5, 106.3205)
  line L580 (37.8397, 106.3205) -> (33.5096, 103.8205)
  line L581 (33.5096, 103.8205) -> (33.5096, 98.8205)
  line L582 (33.5096, 98.8205) -> (37.8397, 96.3205)
  line L583 (37.8397, 96.3205) -> (42.1699, 98.8205)
  line L584 (42.1699, 98.8205) -> (42.1699, 103.8205)
  line L585 (42.1699, 103.8205) -> (37.8397, 106.3205)
  line L586 (27.1795, 106.3205) -> (22.8494, 103.8205)
  line L587 (22.8494, 103.8205) -> (22.8494, 98.8205)
  line L588 (22.8494, 98.8205) -> (27.1795, 96.3205)
  line L589 (27.1795, 96.3205) -> (31.5096, 98.8205)
  line L590 (31.5096, 98.8205) -> (31.5096, 103.8205)
  line L591 (31.5096, 103.8205) -> (27.1795, 106.3205)
  line L592 (16.5192, 106.3205) -> (12.1891, 103.8205)
  line L593 (12.1891, 103.8205) -> (12.1891, 98.8205)
  line L594 (12.1891, 98.8205) -> (16.5192, 96.3205)
  line L595 (16.5192, 96.3205) -> (20.8494, 98.8205)
  line L596 (20.8494, 98.8205) -> (20.8494, 103.8205)
  line L597 (20.8494, 103.8205) -> (16.5192, 106.3205)
  line L598 (5.859, 106.3205) -> (1.5289, 103.8205)
  line L599 (1.5289, 103.8205) -> (1.5289, 98.8205)
  line L600 (1.5289, 98.8205) -> (5.859, 96.3205)
  line L601 (5.859, 96.3205) -> (10.1891, 98.8205)
  line L602 (10.1891, 98.8205) -> (10.1891, 103.8205)
  line L603 (10.1891, 103.8205) -> (5.859, 106.3205)
  line L604 (-4.8013, 106.3205) -> (-9.1314, 103.8205)
  line L605 (-9.1314, 103.8205) -> (-9.1314, 98.8205)
  line L606 (-9.1314, 98.8205) -> (-4.8013, 96.3205)
  line L607 (-4.8013, 96.3205) -> (-0.4711, 98.8205)
  line L608 (-0.4711, 98.8205) -> (-0.4711, 103.8205)
  line L609 (-0.4711, 103.8205) -> (-4.8013, 106.3205)
  line L610 (-15.4615, 106.3205) -> (-19.7917, 103.8205)
  line L611 (-19.7917, 103.8205) -> (-19.7917, 98.8205)
  line L612 (-19.7917, 98.8205) -> (-15.4615, 96.3205)
  line L613 (-15.4615, 96.3205) -> (-11.1314, 98.8205)
  line L614 (-11.1314, 98.8205) -> (-11.1314, 103.8205)
  line L615 (-11.1314, 103.8205) -> (-15.4615, 106.3205)
  line L616 (-26.1218, 106.3205) -> (-30.4519, 103.8205)
  line L617 (-30.4519, 103.8205) -> (-30.4519, 98.8205)
  line L618 (-30.4519, 98.8205) -> (-26.1218, 96.3205)
  line L619 (-26.1218, 96.3205) -> (-21.7917, 98.8205)
  line L620 (-21.7917, 98.8205) -> (-21.7917, 103.8205)
  line L621 (-21.7917, 103.8205) -> (-26.1218, 106.3205)
  line L622 (-36.782, 106.3205) -> (-41.1122, 103.8205)
  line L623 (-41.1122, 103.8205) -> (-41.1122, 98.8205)
  line L624 (-41.1122, 98.8205) -> (-36.782, 96.3205)
  line L625 (-36.782, 96.3205) -> (-32.4519, 98.8205)
  line L626 (-32.4519, 98.8205) -> (-32.4519, 103.8205)
  line L627 (-32.4519, 103.8205) -> (-36.782, 106.3205)
  line L628 (-47.4423, 106.3205) -> (-51.7724, 103.8205)
  line L629 (-51.7724, 103.8205) -> (-51.7724, 98.8205)
  line L630 (-51.7724, 98.8205) -> (-47.4423, 96.3205)
  line L631 (-47.4423, 96.3205) -> (-43.1122, 98.8205)
  line L632 (-43.1122, 98.8205) -> (-43.1122, 103.8205)
  line L633 (-43.1122, 103.8205) -> (-47.4423, 106.3205)
  line L634 (43.1699, 115.5526) -> (38.8397, 113.0526)
  line L635 (38.8397, 113.0526) -> (38.8397, 108.0526)
  line L636 (38.8397, 108.0526) -> (43.1699, 105.5526)
  line L637 (43.1699, 105.5526) -> (47.5, 108.0526)
  line L638 (47.5, 108.0526) -> (47.5, 113.0526)
  line L639 (47.5, 113.0526) -> (43.1699, 115.5526)
  line L640 (32.5096, 115.5526) -> (28.1795, 113.0526)
  line L641 (28.1795, 113.0526) -> (28.1795, 108.0526)
  line L642 (28.1795, 108.0526) -> (32.5096, 105.5526)
  line L643 (32.5096, 105.5526) -> (36.8397, 108.0526)
  line L644 (36.8397, 108.0526) -> (36.8397, 113.0526)
  line L645 (36.8397, 113.0526) -> (32.5096, 115.5526)
  line L646 (21.8494, 115.5526) -> (17.5192, 113.0526)
  line L647 (17.5192, 113.0526) -> (17.5192, 108.0526)
  line L648 (17.5192, 108.0526) -> (21.8494, 105.5526)
  line L649 (21.8494, 105.5526) -> (26.1795, 108.0526)
  line L650 (26.1795, 108.0526) -> (26.1795, 113.0526)
  line L651 (26.1795, 113.0526) -> (21.8494, 115.5526)
  line L652 (11.1891, 115.5526) -> (6.859, 113.0526)
  line L653 (6.859, 113.0526) -> (6.859, 108.0526)
  line L654 (6.859, 108.0526) -> (11.1891, 105.5526)
  line L655 (11.1891, 105.5526) -> (15.5192, 108.0526)
  line L656 (15.5192, 108.0526) -> (15.5192, 113.0526)
  line L657 (15.5192, 113.0526) -> (11.1891, 115.5526)
  line L658 (0.5289, 115.5526) -> (-3.8013, 113.0526)
  line L659 (-3.8013, 113.0526) -> (-3.8013, 108.0526)
  line L660 (-3.8013, 108.0526) -> (0.5289, 105.5526)
  line L661 (0.5289, 105.5526) -> (4.859, 108.0526)
  line L662 (4.859, 108.0526) -> (4.859, 113.0526)
  line L663 (4.859, 113.0526) -> (0.5289, 115.5526)
  line L664 (-10.1314, 115.5526) -> (-14.4615, 113.0526)
  line L665 (-14.4615, 113.0526) -> (-14.4615, 108.0526)
  line L666 (-14.4615, 108.0526) -> (-10.1314, 105.5526)
  line L667 (-10.1314, 105.5526) -> (-5.8013, 108.0526)
  line L668 (-5.8013, 108.0526) -> (-5.8013, 113.0526)
  line L669 (-5.8013, 113.0526) -> (-10.1314, 115.5526)
  line L670 (-20.7917, 115.5526) -> (-25.1218, 113.0526)
  line L671 (-25.1218, 113.0526) -> (-25.1218, 108.0526)
  line L672 (-25.1218, 108.0526) -> (-20.7917, 105.5526)
  line L673 (-20.7917, 105.5526) -> (-16.4615, 108.0526)
  line L674 (-16.4615, 108.0526) -> (-16.4615, 113.0526)
  line L675 (-16.4615, 113.0526) -> (-20.7917, 115.5526)
  line L676 (-31.4519, 115.5526) -> (-35.782, 113.0526)
  line L677 (-35.782, 113.0526) -> (-35.782, 108.0526)
  line L678 (-35.782, 108.0526) -> (-31.4519, 105.5526)
  line L679 (-31.4519, 105.5526) -> (-27.1218, 108.0526)
  line L680 (-27.1218, 108.0526) -> (-27.1218, 113.0526)
  line L681 (-27.1218, 113.0526) -> (-31.4519, 115.5526)
  line L682 (-42.1122, 115.5526) -> (-46.4423, 113.0526)
  line L683 (-46.4423, 113.0526) -> (-46.4423, 108.0526)
  line L684 (-46.4423, 108.0526) -> (-42.1122, 105.5526)
  line L685 (-42.1122, 105.5526) -> (-37.782, 108.0526)
  line L686 (-37.782, 108.0526) -> (-37.782, 113.0526)
  line L687 (-37.782, 113.0526) -> (-42.1122, 115.5526)
  line L688 (48.5, 124.7846) -> (44.1699, 122.2846)
  line L689 (44.1699, 122.2846) -> (44.1699, 117.2846)
  line L690 (44.1699, 117.2846) -> (48.5, 114.7846)
  line L691 (48.5, 114.7846) -> (52.8301, 117.2846)
  line L692 (52.8301, 117.2846) -> (52.8301, 122.2846)
  line L693 (52.8301, 122.2846) -> (48.5, 124.7846)
  line L694 (37.8397, 124.7846) -> (33.5096, 122.2846)
  line L695 (33.5096, 122.2846) -> (33.5096, 117.2846)
  line L696 (33.5096, 117.2846) -> (37.8397, 114.7846)
  line L697 (37.8397, 114.7846) -> (42.1699, 117.2846)
  line L698 (42.1699, 117.2846) -> (42.1699, 122.2846)
  line L699 (42.1699, 122.2846) -> (37.8397, 124.7846)
  line L700 (27.1795, 124.7846) -> (22.8494, 122.2846)
  line L701 (22.8494, 122.2846) -> (22.8494, 117.2846)
  line L702 (22.8494, 117.2846) -> (27.1795, 114.7846)
  line L703 (27.1795, 114.7846) -> (31.5096, 117.2846)
  line L704 (31.5096, 117.2846) -> (31.5096, 122.2846)
  line L705 (31.5096, 122.2846) -> (27.1795, 124.7846)
  line L706 (16.5192, 124.7846) -> (12.1891, 122.2846)
  line L707 (12.1891, 122.2846) -> (12.1891, 117.2846)
  line L708 (12.1891, 117.2846) -> (16.5192, 114.7846)
  line L709 (16.5192, 114.7846) -> (20.8494, 117.2846)
  line L710 (20.8494, 117.2846) -> (20.8494, 122.2846)
  line L711 (20.8494, 122.2846) -> (16.5192, 124.7846)
  line L712 (5.859, 124.7846) -> (1.5289, 122.2846)
  line L713 (1.5289, 122.2846) -> (1.5289, 117.2846)
  line L714 (1.5289, 117.2846) -> (5.859, 114.7846)
  line L715 (5.859, 114.7846) -> (10.1891, 117.2846)
  line L716 (10.1891, 117.2846) -> (10.1891, 122.2846)
  line L717 (10.1891, 122.2846) -> (5.859, 124.7846)
  line L718 (-4.8013, 124.7846) -> (-9.1314, 122.2846)
  line L719 (-9.1314, 122.2846) -> (-9.1314, 117.2846)
  line L720 (-9.1314, 117.2846) -> (-4.8013, 114.7846)
  line L721 (-4.8013, 114.7846) -> (-0.4711, 117.2846)
  line L722 (-0.4711, 117.2846) -> (-0.4711, 122.2846)
  line L723 (-0.4711, 122.2846) -> (-4.8013, 124.7846)
  line L724 (-15.4615, 124.7846) -> (-19.7917, 122.2846)
  line L725 (-19.7917, 122.2846) -> (-19.7917, 117.2846)
  line L726 (-19.7917, 117.2846) -> (-15.4615, 114.7846)
  line L727 (-15.4615, 114.7846) -> (-11.1314, 117.2846)
  line L728 (-11.1314, 117.2846) -> (-11.1314, 122.2846)
  line L729 (-11.1314, 122.2846) -> (-15.4615, 124.7846)
  line L730 (-26.1218, 124.7846) -> (-30.4519, 122.2846)
  line L731 (-30.4519, 122.2846) -> (-30.4519, 117.2846)
  line L732 (-30.4519, 117.2846) -> (-26.1218, 114.7846)
  line L733 (-26.1218, 114.7846) -> (-21.7917, 117.2846)
  line L734 (-21.7917, 117.2846) -> (-21.7917, 122.2846)
  line L735 (-21.7917, 122.2846) -> (-26.1218, 124.7846)
  line L736 (-36.782, 124.7846) -> (-41.1122, 122.2846)
  line L737 (-41.1122, 122.2846) -> (-41.1122, 117.2846)
  line L738 (-41.1122, 117.2846) -> (-36.782, 114.7846)
  line L739 (-36.782, 114.7846) -> (-32.4519, 117.2846)
  line L740 (-32.4519, 117.2846) -> (-32.4519, 122.2846)
  line L741 (-32.4519, 122.2846) -> (-36.782, 124.7846)
  line L742 (-47.4423, 124.7846) -> (-51.7724, 122.2846)
  line L743 (-51.7724, 122.2846) -> (-51.7724, 117.2846)
  line L744 (-51.7724, 117.2846) -> (-47.4423, 114.7846)
  line L745 (-47.4423, 114.7846) -> (-43.1122, 117.2846)
  line L746 (-43.1122, 117.2846) -> (-43.1122, 122.2846)
  line L747 (-43.1122, 122.2846) -> (-47.4423, 124.7846)
  line L748 (43.1699, 134.0167) -> (38.8397, 131.5167)
  line L749 (38.8397, 131.5167) -> (38.8397, 126.5167)
  line L750 (38.8397, 126.5167) -> (43.1699, 124.0167)
  line L751 (43.1699, 124.0167) -> (47.5, 126.5167)
  line L752 (47.5, 126.5167) -> (47.5, 131.5167)
  line L753 (47.5, 131.5167) -> (43.1699, 134.0167)
  line L754 (32.5096, 134.0167) -> (28.1795, 131.5167)
  line L755 (28.1795, 131.5167) -> (28.1795, 126.5167)
  line L756 (28.1795, 126.5167) -> (32.5096, 124.0167)
  line L757 (32.5096, 124.0167) -> (36.8397, 126.5167)
  line L758 (36.8397, 126.5167) -> (36.8397, 131.5167)
  line L759 (36.8397, 131.5167) -> (32.5096, 134.0167)
  line L760 (21.8494, 134.0167) -> (17.5192, 131.5167)
  line L761 (17.5192, 131.5167) -> (17.5192, 126.5167)
  line L762 (17.5192, 126.5167) -> (21.8494, 124.0167)
  line L763 (21.8494, 124.0167) -> (26.1795, 126.5167)
  line L764 (26.1795, 126.5167) -> (26.1795, 131.5167)
  line L765 (26.1795, 131.5167) -> (21.8494, 134.0167)
  line L766 (11.1891, 134.0167) -> (6.859, 131.5167)
  line L767 (6.859, 131.5167) -> (6.859, 126.5167)
  line L768 (6.859, 126.5167) -> (11.1891, 124.0167)
  line L769 (11.1891, 124.0167) -> (15.5192, 126.5167)
  line L770 (15.5192, 126.5167) -> (15.5192, 131.5167)
  line L771 (15.5192, 131.5167) -> (11.1891, 134.0167)
  line L772 (0.5289, 134.0167) -> (-3.8013, 131.5167)
  line L773 (-3.8013, 131.5167) -> (-3.8013, 126.5167)
  line L774 (-3.8013, 126.5167) -> (0.5289, 124.0167)
  line L775 (0.5289, 124.0167) -> (4.859, 126.5167)
  line L776 (4.859, 126.5167) -> (4.859, 131.5167)
  line L777 (4.859, 131.5167) -> (0.5289, 134.0167)
  line L778 (-10.1314, 134.0167) -> (-14.4615, 131.5167)
  line L779 (-14.4615, 131.5167) -> (-14.4615, 126.5167)
  line L780 (-14.4615, 126.5167) -> (-10.1314, 124.0167)
  line L781 (-10.1314, 124.0167) -> (-5.8013, 126.5167)
  line L782 (-5.8013, 126.5167) -> (-5.8013, 131.5167)
  line L783 (-5.8013, 131.5167) -> (-10.1314, 134.0167)
  line L784 (-20.7917, 134.0167) -> (-25.1218, 131.5167)
  line L785 (-25.1218, 131.5167) -> (-25.1218, 126.5167)
  line L786 (-25.1218, 126.5167) -> (-20.7917, 124.0167)
  line L787 (-20.7917, 124.0167) -> (-16.4615, 126.5167)
  line L788 (-16.4615, 126.5167) -> (-16.4615, 131.5167)
  line L789 (-16.4615, 131.5167) -> (-20.7917, 134.0167)
  line L790 (-31.4519, 134.0167) -> (-35.782, 131.5167)
  line L791 (-35.782, 131.5167) -> (-35.782, 126.5167)
  line L792 (-35.782, 126.5167) -> (-31.4519, 124.0167)
  line L793 (-31.4519, 124.0167) -> (-27.1218, 126.5167)
  line L794 (-27.1218, 126.5167) -> (-27.1218, 131.5167)
  line L795 (-27.1218, 131.5167) -> (-31.4519, 134.0167)
  line L796 (-42.1122, 134.0167) -> (-46.4423, 131.5167)
  line L797 (-46.4423, 131.5167) -> (-46.4423, 126.5167)
  line L798 (-46.4423, 126.5167) -> (-42.1122, 124.0167)
  line L799 (-42.1122, 124.0167) -> (-37.782, 126.5167)
  line L800 (-37.782, 126.5167) -> (-37.782, 131.5167)
  line L801 (-37.782, 131.5167) -> (-42.1122, 134.0167)
  line L802 (48.5, 143.2487) -> (44.1699, 140.7487)
  line L803 (44.1699, 140.7487) -> (44.1699, 135.7487)
  line L804 (44.1699, 135.7487) -> (48.5, 133.2487)
  line L805 (48.5, 133.2487) -> (52.8301, 135.7487)
  line L806 (52.8301, 135.7487) -> (52.8301, 140.7487)
  line L807 (52.8301, 140.7487) -> (48.5, 143.2487)
  line L808 (37.8397, 143.2487) -> (33.5096, 140.7487)
  line L809 (33.5096, 140.7487) -> (33.5096, 135.7487)
  line L810 (33.5096, 135.7487) -> (37.8397, 133.2487)
  line L811 (37.8397, 133.2487) -> (42.1699, 135.7487)
  line L812 (42.1699, 135.7487) -> (42.1699, 140.7487)
  line L813 (42.1699, 140.7487) -> (37.8397, 143.2487)
  line L814 (27.1795, 143.2487) -> (22.8494, 140.7487)
  line L815 (22.8494, 140.7487) -> (22.8494, 135.7487)
  line L816 (22.8494, 135.7487) -> (27.1795, 133.2487)
  line L817 (27.1795, 133.2487) -> (31.5096, 135.7487)
  line L818 (31.5096, 135.7487) -> (31.5096, 140.7487)
  line L819 (31.5096, 140.7487) -> (27.1795, 143.2487)
  line L820 (16.5192, 143.2487) -> (12.1891, 140.7487)
  line L821 (12.1891, 140.7487) -> (12.1891, 135.7487)
  line L822 (12.1891, 135.7487) -> (16.5192, 133.2487)
  line L823 (16.5192, 133.2487) -> (20.8494, 135.7487)
  line L824 (20.8494, 135.7487) -> (20.8494, 140.7487)
  line L825 (20.8494, 140.7487) -> (16.5192, 143.2487)
  line L826 (5.859, 143.2487) -> (1.5289, 140.7487)
  line L827 (1.5289, 140.7487) -> (1.5289, 135.7487)
  line L828 (1.5289, 135.7487) -> (5.859, 133.2487)
  line L829 (5.859, 133.2487) -> (10.1891, 135.7487)
  line L830 (10.1891, 135.7487) -> (10.1891, 140.7487)
  line L831 (10.1891, 140.7487) -> (5.859, 143.2487)
  line L832 (-4.8013, 143.2487) -> (-9.1314, 140.7487)
  line L833 (-9.1314, 140.7487) -> (-9.1314, 135.7487)
  line L834 (-9.1314, 135.7487) -> (-4.8013, 133.2487)
  line L835 (-4.8013, 133.2487) -> (-0.4711, 135.7487)
  line L836 (-0.4711, 135.7487) -> (-0.4711, 140.7487)
  line L837 (-0.4711, 140.7487) -> (-4.8013, 143.2487)
  line L838 (-15.4615, 143.2487) -> (-19.7917, 140.7487)
  line L839 (-19.7917, 140.7487) -> (-19.7917, 135.7487)
  line L840 (-19.7917, 135.7487) -> (-15.4615, 133.2487)
  line L841 (-15.4615, 133.2487) -> (-11.1314, 135.7487)
  line L842 (-11.1314, 135.7487) -> (-11.1314, 140.7487)
  line L843 (-11.1314, 140.7487) -> (-15.4615, 143.2487)
  line L844 (-26.1218, 143.2487) -> (-30.4519, 140.7487)
  line L845 (-30.4519, 140.7487) -> (-30.4519, 135.7487)
  line L846 (-30.4519, 135.7487) -> (-26.1218, 133.2487)
  line L847 (-26.1218, 133.2487) -> (-21.7917, 135.7487)
  line L848 (-21.7917, 135.7487) -> (-21.7917, 140.7487)
  line L849 (-21.7917, 140.7487) -> (-26.1218, 143.2487)
  line L850 (-36.782, 143.2487) -> (-41.1122, 140.7487)
  line L851 (-41.1122, 140.7487) -> (-41.1122, 135.7487)
  line L852 (-41.1122, 135.7487) -> (-36.782, 133.2487)
  line L853 (-36.782, 133.2487) -> (-32.4519, 135.7487)
  line L854 (-32.4519, 135.7487) -> (-32.4519, 140.7487)
  line L855 (-32.4519, 140.7487) -> (-36.782, 143.2487)
  line L856 (-47.4423, 143.2487) -> (-51.7724, 140.7487)
  line L857 (-51.7724, 140.7487) -> (-51.7724, 135.7487)
  line L858 (-51.7724, 135.7487) -> (-47.4423, 133.2487)
  line L859 (-47.4423, 133.2487) -> (-43.1122, 135.7487)
  line L860 (-43.1122, 135.7487) -> (-43.1122, 140.7487)
  line L861 (-43.1122, 140.7487) -> (-47.4423, 143.2487)
  line L862 (43.1699, 152.4808) -> (38.8397, 149.9808)
  line L863 (38.8397, 149.9808) -> (38.8397, 144.9808)
  line L864 (38.8397, 144.9808) -> (43.1699, 142.4808)
  line L865 (43.1699, 142.4808) -> (47.5, 144.9808)
  line L866 (47.5, 144.9808) -> (47.5, 149.9808)
  line L867 (47.5, 149.9808) -> (43.1699, 152.4808)
  line L868 (32.5096, 152.4808) -> (28.1795, 149.9808)
  line L869 (28.1795, 149.9808) -> (28.1795, 144.9808)
  line L870 (28.1795, 144.9808) -> (32.5096, 142.4808)
  line L871 (32.5096, 142.4808) -> (36.8397, 144.9808)
  line L872 (36.8397, 144.9808) -> (36.8397, 149.9808)
  line L873 (36.8397, 149.9808) -> (32.5096, 152.4808)
  line L874 (21.8494, 152.4808) -> (17.5192, 149.9808)
  line L875 (17.5192, 149.9808) -> (17.5192, 144.9808)
  line L876 (17.5192, 144.9808) -> (21.8494, 142.4808)
  line L877 (21.8494, 142.4808) -> (26.1795, 144.9808)
  line L878 (26.1795, 144.9808) -> (26.1795, 149.9808)
  line L879 (26.1795, 149.9808) -> (21.8494, 152.4808)
  line L880 (11.1891, 152.4808) -> (6.859, 149.9808)
  line L881 (6.859, 149.9808) -> (6.859, 144.9808)
  line L882 (6.859, 144.9808) -> (11.1891, 142.4808)
  line L883 (11.1891, 142.4808) -> (15.5192, 144.9808)
  line L884 (15.5192, 144.9808) -> (15.5192, 149.9808)
  line L885 (15.5192, 149.9808) -> (11.1891, 152.4808)
  line L886 (0.5289, 152.4808) -> (-3.8013, 149.9808)
  line L887 (-3.8013, 149.9808) -> (-3.8013, 144.9808)
  line L888 (-3.8013, 144.9808) -> (0.5289, 142.4808)
  line L889 (0.5289, 142.4808) -> (4.859, 144.9808)
  line L890 (4.859, 144.9808) -> (4.859, 149.9808)
  line L891 (4.859, 149.9808) -> (0.5289, 152.4808)
  line L892 (-10.1314, 152.4808) -> (-14.4615, 149.9808)
  line L893 (-14.4615, 149.9808) -> (-14.4615, 144.9808)
  line L894 (-14.4615, 144.9808) -> (-10.1314, 142.4808)
  line L895 (-10.1314, 142.4808) -> (-5.8013, 144.9808)
  line L896 (-5.8013, 144.9808) -> (-5.8013, 149.9808)
  line L897 (-5.8013, 149.9808) -> (-10.1314, 152.4808)
  line L898 (-20.7917, 152.4808) -> (-25.1218, 149.9808)
  line L899 (-25.1218, 149.9808) -> (-25.1218, 144.9808)
  line L900 (-25.1218, 144.9808) -> (-20.7917, 142.4808)
  line L901 (-20.7917, 142.4808) -> (-16.4615, 144.9808)